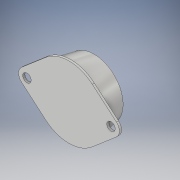
# Autodesk Inventor part: MetallKugellager_V1
Saved by Autodesk Inventor 2017.3 (Build 213257000, 257)
## iProperties
Part Number: MetallKugellager_V1
Material: Generisch
Document SubType Name: Modeling
Designer: Enno-LT
Density: 1 g/cm^3
Appearance: Vorgabe
Author: Enno-LT
Autodesk Inventor part; units mm, degrees
ref_plane "YZ Plane" through (0, 0, 0) normal (1, 0, 0) x (0, 1, 0)
ref_plane "XZ Plane" through (0, 0, 0) normal (0, 1, 0) x (-1, 0, 0)
ref_plane "XY Plane" through (0, 0, 0) normal (0, 0, 1) x (1, 0, 0)
sketch "Skizze2" plane through (0, 0, 0) normal (0, 0, 1) x (1, 0, 0)
  line L0 (-7.07, 14) -> (-8.97, 14)
  line L1 (-8.97, 14) -> (-10.77, 11.3)
  line L2 (-10.77, 11.3) -> (-13.77, 11.3)
  line L3 (-13.77, 11.3) -> (-16, 0)
  line L4 (-16, 0) -> (-15, 0)
  line L5 (-15, 0) -> (-12.9673, 10.3)
  line L6 (-12.9673, 10.3) -> (-10.2348, 10.3)
  line L7 (-10.2348, 10.3) -> (-9.3538, 11.6215)
  line L8 (0, -2.8203) -> (0, 16.9217) projected
  line L9 (-6.4694, 0) -> (0, 0)
  line L10 (0, 0) -> (0, 4)
  line L11 (0, 4) -> (-6.4694, 4)
  line L12 (-6.4694, 4) -> (-6.4694, 0)
  arc A0 (-7.07, 14) -> (-9.3538, 11.6215) centre (-1.5666, 6.43) ccw
  point P0 (-15.5, 0)
  point P1 (-3.2347, 0)
  dimension "d1" = 14
  dimension "d2" = 1.9
  dimension "d5" = 1.8
  dimension "d8" = 1
  dimension "d9" = 1
  dimension "d10" = 1
  dimension "d15" = 2.7
  dimension "d52" = 7.07
  dimension "d53" = 10
  dimension "d54" = 6.4694
  dimension "d58" = 9.3591
  dimension "d60" = 16
  dimension "d61" = 3
  constraints: 24 end point, 5 parallel, 4 horizontal, 2 horizontal alignment, 2 midpoint, 2 point on circle, 1 centre point, 1 perpendicular, 1 point on line, 1 tangent
  measures "d1" distance between parallel lines of L4 L0
  measures "d2" distance of L0.start L0.end
  measures "d5" horizontal distance of L1.end L0.end
  measures "d8" distance of L3.end L4.end
  measures "d9" distance between parallel lines of L2 L6
  measures "d10" distance between parallel lines of L7 L1
  measures "d15" distance between parallel lines of L2 L0
  measures "d52" distance from line of L8 L0.start
  measures "d53" distance from line of L0.start L11
  measures "d54" distance of L10.end L11.end
  measures "d58" radius of A0
  measures "d60" distance of L9.end L3.end
  measures "d61" distance of L1.end L2.end
revolve "Umdrehung1" add sketch "Skizze2" angle 360 about axis through (0, -10, 0) along (0, 1, 0)
sketch "Skizze3" plane through (0, 0, 0) normal (0, 1, 0) x (-1, 0, 0)
  circle A0 centre (20, 0) radius 2
  circle A1 centre (-20, 0) radius 2
  circle A2 centre (0, 0) radius 16 construction
  arc A3 (22.6, -3.0397) -> (22.6, 3.0397) centre (20, 0) ccw
  arc A4 (-22.6, 3.0397) -> (-22.6, -3.0397) centre (-20, 0) ccw
  line L0 (22.6, -3.0397) -> (11.05, -12.9189)
  line L1 (22.6, -3.0397) -> (22.6, 13.4844) construction
  line L2 (22.6, 3.0397) -> (11.05, 12.9189)
  line L3 (-11.05, 12.9189) -> (-22.6, 3.0397)
  line L4 (-22.6, -3.0397) -> (-11.05, -12.9189)
  arc A5 (11.05, 12.9189) -> (-11.05, 12.9189) centre (0, 0) ccw
  arc A6 (-11.05, -12.9189) -> (11.05, -12.9189) centre (0, 0) ccw
  line L5 (0, -19.9813) -> (0, 17.4256) construction
  circle A7 centre (0, 0) radius 17 construction
  point P0 (0, -17)
  point P1 (0, 17)
  dimension "d32" = 36
  dimension "d33" = 40
  dimension "d34" = 20
  dimension "d36" = 4
  dimension "d37" = 8
  dimension "d38" = 8
  dimension "d39" = 4
  dimension "d42" = 1
  constraints: 12 end point, 10 point on circle, 7 tangent, 6 centre point, 5 coincident, 3 point on line, 2 horizontal alignment, 2 line through centre, 2 vertical, 1 vertical alignment, 2 other
  measures "d33" distance of A0.centre A1.centre
  measures "d34" distance of point (0, 0) A0.centre
  measures "d36" diameter of A0
  measures "d37" diameter of A4
  measures "d38" diameter of A3
  measures "d39" diameter of A1
extrude "Extrusion1" add sketch "Skizze3" against normal blind 1
sketch "Skizze4" plane through (0, 0, 0) normal (0, 0, 1) x (1, 0, 0)
  arc A0 (0, 19) -> (0, 4) centre (0, 11.5) ccw
  line L0 (7.07, 14) -> (-7.07, 14) projected
  line L1 (0, 4) -> (-20.7674, 4) construction
  line L2 (0, 19) -> (0, 4)
  point P0 (0, 0)
  point P1 (0, 11.5)
  dimension "d45" = 15
  dimension "d46" = 5
  constraints: 4 end point, 2 point on circle, 1 centre point, 1 horizontal, 1 midpoint, 1 tangent, 1 vertical, 1 vertical alignment
  measures "d45" diameter of A0
  measures "d46" distance edge to line of A0 L0
revolve "Umdrehung2" add sketch "Skizze4" angle 360 about axis through (0, 19, 0) along (0, -1, 0)
fillet "Rundung1" radius 0.5 4 edges at (8.97, 14, 0) (10.77, 11.3, 0) (13.77, 11.3, 0) (16, 0, 0)
